AnimationGear v7 (Autodesk Fusion 360 design; units mm, degrees)
Autodesk Fusion 360 part; units mm, degrees
note: some values were not read from the file. Set by a fixed rule: which sketch regions a step uses.
sketch "Sketch1" plane through (0, 0, 0) normal (0, 1, 0) x (1, 0, 0)
  line L0 (7.1438, 0) -> (11.7891, 0)
  line L1 (11.7891, 0) -> (11.8321, 0.0026)
  line L2 (11.8321, 0.0026) -> (11.9318, 0.0152)
  line L3 (11.9318, 0.0152) -> (12.0868, 0.0457)
  line L4 (12.0868, 0.0457) -> (12.2948, 0.1017)
  line L5 (12.2948, 0.1017) -> (12.5526, 0.1909)
  line L6 (12.5526, 0.1909) -> (12.8565, 0.3202)
  line L7 (12.8565, 0.3202) -> (13.2018, 0.4965)
  line L8 (13.2018, 0.4965) -> (13.5832, 0.7261)
  line L9 (13.5832, 0.7261) -> (13.9947, 1.0146)
  line L10 (13.9947, 1.0146) -> (14.4297, 1.3673)
  line L11 (14.4297, 1.3673) -> (14.881, 1.7887)
  line L12 (14.881, 1.7887) -> (15.3411, 2.2825)
  line L13 (15.3411, 2.2825) -> (15.8017, 2.8518)
  line L14 (15.8017, 2.8518) -> (16.2544, 3.499)
  line L15 (16.2544, 3.499) -> (16.6905, 4.2253)
  line L16 (16.6905, 4.2253) -> (17.1009, 5.0316)
  line L17 (17.1009, 5.0316) -> (17.4765, 5.9173)
  line L18 (17.4765, 5.9173) -> (17.1551, 6.7931)
  line L19 (17.1551, 6.7931) -> (16.2957, 7.2255)
  line L20 (16.2957, 7.2255) -> (15.4612, 7.5748)
  line L21 (15.4612, 7.5748) -> (14.6587, 7.8467)
  line L22 (14.6587, 7.8467) -> (13.8949, 8.0473)
  line L23 (13.8949, 8.0473) -> (13.1753, 8.1835)
  line L24 (13.1753, 8.1835) -> (12.5051, 8.2625)
  line L25 (12.5051, 8.2625) -> (11.8883, 8.2918)
  line L26 (11.8883, 8.2918) -> (11.3284, 8.2793)
  line L27 (11.3284, 8.2793) -> (10.828, 8.2332)
  line L28 (10.828, 8.2332) -> (10.3886, 8.1615)
  line L29 (10.3886, 8.1615) -> (10.0113, 8.0726)
  line L30 (10.0113, 8.0726) -> (9.6958, 7.9747)
  line L31 (9.6958, 7.9747) -> (9.4415, 7.8758)
  line L32 (9.4415, 7.8758) -> (9.2467, 7.7841)
  line L33 (9.2467, 7.7841) -> (9.1088, 7.707)
  line L34 (9.1088, 7.707) -> (9.0246, 7.6521)
  line L35 (9.0246, 7.6521) -> (8.9901, 7.6263)
  line L36 (8.9901, 7.6263) -> (5.4477, 4.6213)
  line L37 (5.4477, 4.6213) -> (2.2076, 6.7941)
  line L38 (2.2076, 6.7941) -> (3.643, 11.2121)
  line L39 (3.643, 11.2121) -> (3.6538, 11.2538)
  line L40 (3.6538, 11.2538) -> (3.6727, 11.3525)
  line L41 (3.6727, 11.3525) -> (3.6916, 11.5093)
  line L42 (3.6916, 11.5093) -> (3.7025, 11.7244)
  line L43 (3.7025, 11.7244) -> (3.6974, 11.9972)
  line L44 (3.6974, 11.9972) -> (3.6683, 12.3262)
  line L45 (3.6683, 12.3262) -> (3.6074, 12.7091)
  line L46 (3.6074, 12.7091) -> (3.5069, 13.1428)
  line L47 (3.5069, 13.1428) -> (3.3596, 13.6233)
  line L48 (3.3596, 13.6233) -> (3.1586, 14.146)
  line L49 (3.1586, 14.146) -> (2.8974, 14.7054)
  line L50 (2.8974, 14.7054) -> (2.5699, 15.2956)
  line L51 (2.5699, 15.2956) -> (2.1707, 15.9096)
  line L52 (2.1707, 15.9096) -> (1.6952, 16.5401)
  line L53 (1.6952, 16.5401) -> (1.1391, 17.1793)
  line L54 (1.1391, 17.1793) -> (0.4992, 17.8187)
  line L55 (0.4992, 17.8187) -> (-0.2271, 18.4497)
  line L56 (-0.2271, 18.4497) -> (-1.1594, 18.4146)
  line L57 (-1.1594, 18.4146) -> (-1.8362, 17.7309)
  line L58 (-1.8362, 17.7309) -> (-2.4263, 17.0452)
  line L59 (-2.4263, 17.0452) -> (-2.9328, 16.366)
  line L60 (-2.9328, 16.366) -> (-3.3597, 15.7016)
  line L61 (-3.3597, 15.7016) -> (-3.7115, 15.0593)
  line L62 (-3.7115, 15.0593) -> (-3.9938, 14.4463)
  line L63 (-3.9938, 14.4463) -> (-4.2123, 13.8687)
  line L64 (-4.2123, 13.8687) -> (-4.3735, 13.3324)
  line L65 (-4.3735, 13.3324) -> (-4.4842, 12.8422)
  line L66 (-4.4842, 12.8422) -> (-4.5518, 12.4022)
  line L67 (-4.5518, 12.4022) -> (-4.5839, 12.0158)
  line L68 (-4.5839, 12.0158) -> (-4.5882, 11.6856)
  line L69 (-4.5882, 11.6856) -> (-4.5728, 11.4132)
  line L70 (-4.5728, 11.4132) -> (-4.5457, 11.1995)
  line L71 (-4.5457, 11.1995) -> (-4.5151, 11.0446)
  line L72 (-4.5151, 11.0446) -> (-4.4888, 10.9475)
  line L73 (-4.4888, 10.9475) -> (-4.4749, 10.9068)
  line L74 (-4.4749, 10.9068) -> (-2.7117, 6.6091)
  line L75 (-2.7117, 6.6091) -> (-5.7794, 4.199)
  line L76 (-5.7794, 4.199) -> (-9.5376, 6.9294)
  line L77 (-9.5376, 6.9294) -> (-9.5739, 6.9526)
  line L78 (-9.5739, 6.9526) -> (-9.6619, 7.001)
  line L79 (-9.6619, 7.001) -> (-9.8052, 7.0675)
  line L80 (-9.8052, 7.0675) -> (-10.0065, 7.1444)
  line L81 (-10.0065, 7.1444) -> (-10.2675, 7.2238)
  line L82 (-10.2675, 7.2238) -> (-10.5893, 7.2978)
  line L83 (-10.5893, 7.2978) -> (-10.9723, 7.3581)
  line L84 (-10.9723, 7.3581) -> (-11.4158, 7.3966)
  line L85 (-11.4158, 7.3966) -> (-11.9183, 7.405)
  line L86 (-11.9183, 7.405) -> (-12.4776, 7.3754)
  line L87 (-12.4776, 7.3754) -> (-13.0904, 7.2998)
  line L88 (-13.0904, 7.2998) -> (-13.7528, 7.1707)
  line L89 (-13.7528, 7.1707) -> (-14.4601, 6.9808)
  line L90 (-14.4601, 6.9808) -> (-15.2067, 6.7234)
  line L91 (-15.2067, 6.7234) -> (-15.9865, 6.392)
  line L92 (-15.9865, 6.392) -> (-16.7924, 5.981)
  line L93 (-16.7924, 5.981) -> (-17.6169, 5.4852)
  line L94 (-17.6169, 5.4852) -> (-17.8716, 4.5878)
  line L95 (-17.8716, 4.5878) -> (-17.4305, 3.7328)
  line L96 (-17.4305, 3.7328) -> (-16.9607, 2.9597)
  line L97 (-16.9607, 2.9597) -> (-16.4713, 2.2681)
  line L98 (-16.4713, 2.2681) -> (-15.9713, 1.6568)
  line L99 (-15.9713, 1.6568) -> (-15.4692, 1.1237)
  line L100 (-15.4692, 1.1237) -> (-14.9734, 0.6658)
  line L101 (-14.9734, 0.6658) -> (-14.4916, 0.2796)
  line L102 (-14.4916, 0.2796) -> (-14.0314, -0.0395)
  line L103 (-14.0314, -0.0395) -> (-13.5993, -0.2963)
  line L104 (-13.5993, -0.2963) -> (-13.2018, -0.4965)
  line L105 (-13.2018, -0.4965) -> (-12.8442, -0.6464)
  line L106 (-12.8442, -0.6464) -> (-12.5315, -0.7526)
  line L107 (-12.5315, -0.7526) -> (-12.2677, -0.8221)
  line L108 (-12.2677, -0.8221) -> (-12.0561, -0.8624)
  line L109 (-12.0561, -0.8624) -> (-11.8992, -0.8811)
  line L110 (-11.8992, -0.8811) -> (-11.7988, -0.8862)
  line L111 (-11.7988, -0.8862) -> (-11.7558, -0.8855)
  line L112 (-11.7558, -0.8855) -> (-7.1236, -0.5366)
  line L113 (-7.1236, -0.5366) -> (-5.7794, -4.199)
  line L114 (-5.7794, -4.199) -> (-9.5375, -6.9295)
  line L115 (-9.5375, -6.9295) -> (-9.5708, -6.9568)
  line L116 (-9.5708, -6.9568) -> (-9.6441, -7.0256)
  line L117 (-9.6441, -7.0256) -> (-9.7516, -7.1414)
  line L118 (-9.7516, -7.1414) -> (-9.8869, -7.309)
  line L119 (-9.8869, -7.309) -> (-10.0431, -7.5327)
  line L120 (-10.0431, -7.5327) -> (-10.2129, -7.8159)
  line L121 (-10.2129, -7.8159) -> (-10.3886, -8.1615)
  line L122 (-10.3886, -8.1615) -> (-10.5622, -8.5714)
  line L123 (-10.5622, -8.5714) -> (-10.7255, -9.0467)
  line L124 (-10.7255, -9.0467) -> (-10.8702, -9.5878)
  line L125 (-10.8702, -9.5878) -> (-10.9877, -10.1939)
  line L126 (-10.9877, -10.1939) -> (-11.0696, -10.8638)
  line L127 (-11.0696, -10.8638) -> (-11.1076, -11.5952)
  line L128 (-11.1076, -11.5952) -> (-11.0935, -12.3848)
  line L129 (-11.0935, -12.3848) -> (-11.0193, -13.2288)
  line L130 (-11.0193, -13.2288) -> (-10.8774, -14.1222)
  line L131 (-10.8774, -14.1222) -> (-10.6607, -15.0596)
  line L132 (-10.6607, -15.0596) -> (-9.8859, -15.5792)
  line L133 (-9.8859, -15.5792) -> (-8.9364, -15.4239)
  line L134 (-8.9364, -15.4239) -> (-8.056, -15.216)
  line L135 (-8.056, -15.216) -> (-7.247, -14.9643)
  line L136 (-7.247, -14.9643) -> (-6.5111, -14.6776)
  line L137 (-6.5111, -14.6776) -> (-5.8489, -14.3648)
  line L138 (-5.8489, -14.3648) -> (-5.2603, -14.0348)
  line L139 (-5.2603, -14.0348) -> (-4.744, -13.696)
  line L140 (-4.744, -13.696) -> (-4.2984, -13.3568)
  line L141 (-4.2984, -13.3568) -> (-3.9206, -13.0253)
  line L142 (-3.9206, -13.0253) -> (-3.6074, -12.7091)
  line L143 (-3.6074, -12.7091) -> (-3.3543, -12.4153)
  line L144 (-3.3543, -12.4153) -> (-3.1567, -12.1507)
  line L145 (-3.1567, -12.1507) -> (-3.0091, -11.9213)
  line L146 (-3.0091, -11.9213) -> (-2.9054, -11.7325)
  line L147 (-2.9054, -11.7325) -> (-2.8391, -11.5891)
  line L148 (-2.8391, -11.5891) -> (-2.8032, -11.4952)
  line L149 (-2.8032, -11.4952) -> (-2.7905, -11.4541)
  line L150 (-2.7905, -11.4541) -> (-1.691, -6.9407)
  line L151 (-1.691, -6.9407) -> (2.2076, -6.7941)
  line L152 (2.2076, -6.7941) -> (3.643, -11.2121)
  line L153 (3.643, -11.2121) -> (3.6588, -11.2522)
  line L154 (3.6588, -11.2522) -> (3.7016, -11.3431)
  line L155 (3.7016, -11.3431) -> (3.7784, -11.4811)
  line L156 (3.7784, -11.4811) -> (3.896, -11.6616)
  line L157 (3.896, -11.6616) -> (4.0605, -11.8793)
  line L158 (4.0605, -11.8793) -> (4.2774, -12.1283)
  line L159 (4.2774, -12.1283) -> (4.5518, -12.4022)
  line L160 (4.5518, -12.4022) -> (4.888, -12.694)
  line L161 (4.888, -12.694) -> (5.2896, -12.9962)
  line L162 (5.2896, -12.9962) -> (5.7594, -13.3009)
  line L163 (5.7594, -13.3009) -> (6.2996, -13.6)
  line L164 (6.2996, -13.6) -> (6.9114, -13.8849)
  line L165 (6.9114, -13.8849) -> (7.5953, -14.147)
  line L166 (7.5953, -14.147) -> (8.3506, -14.3776)
  line L167 (8.3506, -14.3776) -> (9.1762, -14.5679)
  line L168 (9.1762, -14.5679) -> (10.0698, -14.7091)
  line L169 (10.0698, -14.7091) -> (11.0282, -14.7926)
  line L170 (11.0282, -14.7926) -> (11.7618, -14.2163)
  line L171 (11.7618, -14.2163) -> (11.9075, -13.2653)
  line L172 (11.9075, -13.2653) -> (11.9818, -12.3637)
  line L173 (11.9818, -12.3637) -> (11.9924, -11.5165)
  line L174 (11.9924, -11.5165) -> (11.9472, -10.7281)
  line L175 (11.9472, -10.7281) -> (11.8544, -10.0016)
  line L176 (11.8544, -10.0016) -> (11.7223, -9.3398)
  line L177 (11.7223, -9.3398) -> (11.5596, -8.7441)
  line L178 (11.5596, -8.7441) -> (11.3748, -8.2155)
  line L179 (11.3748, -8.2155) -> (11.1763, -7.7538)
  line L180 (11.1763, -7.7538) -> (10.9723, -7.3581)
  line L181 (10.9723, -7.3581) -> (10.7712, -7.0267)
  line L182 (10.7712, -7.0267) -> (10.5805, -6.757)
  line L183 (10.5805, -6.757) -> (10.408, -6.5457)
  line L184 (10.408, -6.5457) -> (10.2605, -6.3887)
  line L185 (10.2605, -6.3887) -> (10.1446, -6.2813)
  line L186 (10.1446, -6.2813) -> (10.0663, -6.2182)
  line L187 (10.0663, -6.2182) -> (10.0311, -6.1934)
  line L188 (10.0311, -6.1934) -> (6.0785, -3.753)
  line L189 (6.0785, -3.753) -> (7.1438, 0)
  line L190 (2.6458, 0) -> (-2.6458, 0)
  line L191 (0, -2.6458) -> (0, 2.6458)
  circle A0 centre (12.4191, 4.558) radius 2.077
  circle A1 centre (0, 0) radius 13.2292
  circle A2 centre (0, 0) radius 18.5208
  circle A3 centre (0, 0) radius 11.7872
  circle A4 centre (0, 0) radius 1.5
  dimension "d1" = 3
  constraint concentric A2 A4
  measures "d1" diameter of A4
extrude "Extrude1" add sketch "Sketch1" along normal blind 5 contours L0 L36 L37 L38 L74 L75 L76 L112 L113 L114 L150 L151 L152 L188 L189 A0 A3 | L1 L2 L3 L4 L5 L6 L7 L8 A0 A1 A3 | L153 L154 L155 L156 L157 L158 L159 L160 L180 L181 L182 L183 L184 L185 L186 L187 A1 A3 | A0 A1 A3 | A0 A3 | L28 L29 L30 L31 L32 L33 L34 L35 A0 A1 A3 | A0 A1 | L8 L9 L10 L11 L12 L13 L14 L15 L16 L17 L18 L19 L20 L21 L22 L23 L24 L25 L26 L27 L28 A0 A1 | L115 L116 L117 L118 L119 L120 L121 L122 L142 L143 L144 L145 L146 L147 L148 L149 A1 A3 | L39 L40 L41 L42 L43 L44 L45 L46 L66 L67 L68 L69 L70 L71 L72 L73 A1 A3 | L77 L78 L79 L80 L81 L82 L83 L84 L104 L105 L106 L107 L108 L109 L110 L111 A1 A3 | L46 L47 L48 L49 L50 L51 L52 L53 L54 L55 L56 L57 L58 L59 L60 L61 L62 L63 L64 L65 L66 A1 | L160 L161 L162 L163 L164 L165 L166 L167 L168 L169 L170 L171 L172 L173 L174 L175 L176 L177 L178 L179 L180 A1 | L84 L85 L86 L87 L88 L89 L90 L91 L92 L93 L94 L95 L96 L97 L98 L99 L100 L101 L102 L103 L104 A1 | L122 L123 L124 L125 L126 L127 L128 L129 L130 L131 L132 L133 L134 L135 L136 L137 L138 L139 L140 L141 L142 A1
sketch "Sketch2" plane through (0, 5, 0) normal (0, 1, 0) x (-1, 0, 0)
  circle A0 centre (0, 0) radius 1.5
  line L0 (-6.0785, 3.753) -> (-7.1438, 0)
  line L1 (-7.1438, 0) -> (-11.7891, 0)
  line L2 (-11.7891, 0) -> (-11.8321, -0.0026)
  line L3 (-11.8321, -0.0026) -> (-11.9318, -0.0152)
  line L4 (-11.9318, -0.0152) -> (-12.0868, -0.0457)
  line L5 (-12.0868, -0.0457) -> (-12.2948, -0.1017)
  line L6 (-12.2948, -0.1017) -> (-12.5526, -0.1909)
  line L7 (-12.5526, -0.1909) -> (-12.8565, -0.3202)
  line L8 (-12.8565, -0.3202) -> (-13.2018, -0.4965)
  line L9 (-13.2018, -0.4965) -> (-13.5832, -0.7261)
  line L10 (-13.5832, -0.7261) -> (-13.9947, -1.0146)
  line L11 (-13.9947, -1.0146) -> (-14.4297, -1.3673)
  line L12 (-14.4297, -1.3673) -> (-14.881, -1.7887)
  line L13 (-14.881, -1.7887) -> (-15.3411, -2.2825)
  line L14 (-15.3411, -2.2825) -> (-15.8017, -2.8518)
  line L15 (-15.8017, -2.8518) -> (-16.2544, -3.499)
  line L16 (-16.2544, -3.499) -> (-16.6905, -4.2253)
  line L17 (-16.6905, -4.2253) -> (-17.1009, -5.0316)
  line L18 (-17.1009, -5.0316) -> (-17.4765, -5.9173)
  line L19 (-17.4765, -5.9173) -> (-17.1551, -6.7931)
  line L20 (-17.1551, -6.7931) -> (-16.2957, -7.2255)
  line L21 (-16.2957, -7.2255) -> (-15.4612, -7.5748)
  line L22 (-15.4612, -7.5748) -> (-14.6587, -7.8467)
  line L23 (-14.6587, -7.8467) -> (-13.8949, -8.0473)
  line L24 (-13.8949, -8.0473) -> (-13.1753, -8.1835)
  line L25 (-13.1753, -8.1835) -> (-12.5051, -8.2625)
  line L26 (-12.5051, -8.2625) -> (-11.8883, -8.2918)
  line L27 (-11.8883, -8.2918) -> (-11.3284, -8.2793)
  line L28 (-11.3284, -8.2793) -> (-10.828, -8.2332)
  line L29 (-10.828, -8.2332) -> (-10.3886, -8.1615)
  line L30 (-10.3886, -8.1615) -> (-10.0113, -8.0726)
  line L31 (-10.0113, -8.0726) -> (-9.6958, -7.9747)
  line L32 (-9.6958, -7.9747) -> (-9.4415, -7.8758)
  line L33 (-9.4415, -7.8758) -> (-9.2467, -7.7841)
  line L34 (-9.2467, -7.7841) -> (-9.1088, -7.707)
  line L35 (-9.1088, -7.707) -> (-9.0246, -7.6521)
  line L36 (-9.0246, -7.6521) -> (-8.9901, -7.6263)
  line L37 (-8.9901, -7.6263) -> (-5.4477, -4.6213)
  line L38 (-5.4477, -4.6213) -> (-2.2076, -6.7941)
  line L39 (-2.2076, -6.7941) -> (-3.643, -11.2121)
  line L40 (-3.643, -11.2121) -> (-3.6538, -11.2538)
  line L41 (-3.6538, -11.2538) -> (-3.6727, -11.3525)
  line L42 (-3.6727, -11.3525) -> (-3.6916, -11.5093)
  line L43 (-3.6916, -11.5093) -> (-3.7025, -11.7244)
  line L44 (-3.7025, -11.7244) -> (-3.6974, -11.9972)
  line L45 (-3.6974, -11.9972) -> (-3.6683, -12.3262)
  line L46 (-3.6683, -12.3262) -> (-3.6074, -12.7091)
  line L47 (-3.6074, -12.7091) -> (-3.5069, -13.1428)
  line L48 (-3.5069, -13.1428) -> (-3.3596, -13.6233)
  line L49 (-3.3596, -13.6233) -> (-3.1586, -14.146)
  line L50 (-3.1586, -14.146) -> (-2.8974, -14.7054)
  line L51 (-2.8974, -14.7054) -> (-2.5699, -15.2956)
  line L52 (-2.5699, -15.2956) -> (-2.1707, -15.9096)
  line L53 (-2.1707, -15.9096) -> (-1.6952, -16.5401)
  line L54 (-1.6952, -16.5401) -> (-1.1391, -17.1793)
  line L55 (-1.1391, -17.1793) -> (-0.4992, -17.8187)
  line L56 (-0.4992, -17.8187) -> (0.2271, -18.4497)
  line L57 (0.2271, -18.4497) -> (1.1594, -18.4146)
  line L58 (1.1594, -18.4146) -> (1.8362, -17.7309)
  line L59 (1.8362, -17.7309) -> (2.4263, -17.0452)
  line L60 (2.4263, -17.0452) -> (2.9328, -16.366)
  line L61 (2.9328, -16.366) -> (3.3597, -15.7016)
  line L62 (3.3597, -15.7016) -> (3.7115, -15.0593)
  line L63 (3.7115, -15.0593) -> (3.9938, -14.4463)
  line L64 (3.9938, -14.4463) -> (4.2123, -13.8687)
  line L65 (4.2123, -13.8687) -> (4.3735, -13.3324)
  line L66 (4.3735, -13.3324) -> (4.4842, -12.8422)
  line L67 (4.4842, -12.8422) -> (4.5518, -12.4022)
  line L68 (4.5518, -12.4022) -> (4.5839, -12.0158)
  line L69 (4.5839, -12.0158) -> (4.5882, -11.6856)
  line L70 (4.5882, -11.6856) -> (4.5728, -11.4132)
  line L71 (4.5728, -11.4132) -> (4.5457, -11.1995)
  line L72 (4.5457, -11.1995) -> (4.5151, -11.0446)
  line L73 (4.5151, -11.0446) -> (4.4888, -10.9475)
  line L74 (4.4888, -10.9475) -> (4.4749, -10.9068)
  line L75 (4.4749, -10.9068) -> (2.7117, -6.6091)
  line L76 (2.7117, -6.6091) -> (5.7794, -4.199)
  line L77 (5.7794, -4.199) -> (9.5376, -6.9294)
  line L78 (9.5376, -6.9294) -> (9.5739, -6.9526)
  line L79 (9.5739, -6.9526) -> (9.6619, -7.001)
  line L80 (9.6619, -7.001) -> (9.8052, -7.0675)
  line L81 (9.8052, -7.0675) -> (10.0065, -7.1444)
  line L82 (10.0065, -7.1444) -> (10.2675, -7.2238)
  line L83 (10.2675, -7.2238) -> (10.5893, -7.2978)
  line L84 (10.5893, -7.2978) -> (10.9723, -7.3581)
  line L85 (10.9723, -7.3581) -> (11.4158, -7.3966)
  line L86 (11.4158, -7.3966) -> (11.9183, -7.405)
  line L87 (11.9183, -7.405) -> (12.4776, -7.3754)
  line L88 (12.4776, -7.3754) -> (13.0904, -7.2998)
  line L89 (13.0904, -7.2998) -> (13.7528, -7.1707)
  line L90 (13.7528, -7.1707) -> (14.4601, -6.9808)
  line L91 (14.4601, -6.9808) -> (15.2067, -6.7234)
  line L92 (15.2067, -6.7234) -> (15.9865, -6.392)
  line L93 (15.9865, -6.392) -> (16.7924, -5.981)
  line L94 (16.7924, -5.981) -> (17.6169, -5.4852)
  line L95 (17.6169, -5.4852) -> (17.8716, -4.5878)
  line L96 (17.8716, -4.5878) -> (17.4305, -3.7328)
  line L97 (17.4305, -3.7328) -> (16.9607, -2.9597)
  line L98 (16.9607, -2.9597) -> (16.4713, -2.2681)
  line L99 (16.4713, -2.2681) -> (15.9713, -1.6568)
  line L100 (15.9713, -1.6568) -> (15.4692, -1.1237)
  line L101 (15.4692, -1.1237) -> (14.9734, -0.6658)
  line L102 (14.9734, -0.6658) -> (14.4916, -0.2796)
  line L103 (14.4916, -0.2796) -> (14.0314, 0.0395)
  line L104 (14.0314, 0.0395) -> (13.5993, 0.2963)
  line L105 (13.5993, 0.2963) -> (13.2018, 0.4965)
  line L106 (13.2018, 0.4965) -> (12.8442, 0.6464)
  line L107 (12.8442, 0.6464) -> (12.5315, 0.7526)
  line L108 (12.5315, 0.7526) -> (12.2677, 0.8221)
  line L109 (12.2677, 0.8221) -> (12.0561, 0.8624)
  line L110 (12.0561, 0.8624) -> (11.8992, 0.8811)
  line L111 (11.8992, 0.8811) -> (11.7988, 0.8862)
  line L112 (11.7988, 0.8862) -> (11.7558, 0.8855)
  line L113 (11.7558, 0.8855) -> (7.1236, 0.5366)
  line L114 (7.1236, 0.5366) -> (5.7794, 4.199)
  line L115 (5.7794, 4.199) -> (9.5375, 6.9295)
  line L116 (9.5375, 6.9295) -> (9.5708, 6.9568)
  line L117 (9.5708, 6.9568) -> (9.6441, 7.0256)
  line L118 (9.6441, 7.0256) -> (9.7516, 7.1414)
  line L119 (9.7516, 7.1414) -> (9.8869, 7.309)
  line L120 (9.8869, 7.309) -> (10.0431, 7.5327)
  line L121 (10.0431, 7.5327) -> (10.2129, 7.8159)
  line L122 (10.2129, 7.8159) -> (10.3886, 8.1615)
  line L123 (10.3886, 8.1615) -> (10.5622, 8.5714)
  line L124 (10.5622, 8.5714) -> (10.7255, 9.0467)
  line L125 (10.7255, 9.0467) -> (10.8702, 9.5878)
  line L126 (10.8702, 9.5878) -> (10.9877, 10.1939)
  line L127 (10.9877, 10.1939) -> (11.0696, 10.8638)
  line L128 (11.0696, 10.8638) -> (11.1076, 11.5952)
  line L129 (11.1076, 11.5952) -> (11.0935, 12.3848)
  line L130 (11.0935, 12.3848) -> (11.0193, 13.2288)
  line L131 (11.0193, 13.2288) -> (10.8774, 14.1222)
  line L132 (10.8774, 14.1222) -> (10.6607, 15.0596)
  line L133 (10.6607, 15.0596) -> (9.8859, 15.5792)
  line L134 (9.8859, 15.5792) -> (8.9364, 15.4239)
  line L135 (8.9364, 15.4239) -> (8.056, 15.216)
  line L136 (8.056, 15.216) -> (7.247, 14.9643)
  line L137 (7.247, 14.9643) -> (6.5111, 14.6776)
  line L138 (6.5111, 14.6776) -> (5.8489, 14.3648)
  line L139 (5.8489, 14.3648) -> (5.2603, 14.0348)
  line L140 (5.2603, 14.0348) -> (4.744, 13.696)
  line L141 (4.744, 13.696) -> (4.2984, 13.3568)
  line L142 (4.2984, 13.3568) -> (3.9206, 13.0253)
  line L143 (3.9206, 13.0253) -> (3.6074, 12.7091)
  line L144 (3.6074, 12.7091) -> (3.3543, 12.4153)
  line L145 (3.3543, 12.4153) -> (3.1567, 12.1507)
  line L146 (3.1567, 12.1507) -> (3.0091, 11.9213)
  line L147 (3.0091, 11.9213) -> (2.9054, 11.7325)
  line L148 (2.9054, 11.7325) -> (2.8391, 11.5891)
  line L149 (2.8391, 11.5891) -> (2.8032, 11.4952)
  line L150 (2.8032, 11.4952) -> (2.7905, 11.4541)
  line L151 (2.7905, 11.4541) -> (1.691, 6.9407)
  line L152 (1.691, 6.9407) -> (-2.2076, 6.7941)
  line L153 (-2.2076, 6.7941) -> (-3.643, 11.2121)
  line L154 (-3.643, 11.2121) -> (-3.6588, 11.2522)
  line L155 (-3.6588, 11.2522) -> (-3.7016, 11.3431)
  line L156 (-3.7016, 11.3431) -> (-3.7784, 11.4811)
  line L157 (-3.7784, 11.4811) -> (-3.896, 11.6616)
  line L158 (-3.896, 11.6616) -> (-4.0605, 11.8793)
  line L159 (-4.0605, 11.8793) -> (-4.2774, 12.1283)
  line L160 (-4.2774, 12.1283) -> (-4.5518, 12.4022)
  line L161 (-4.5518, 12.4022) -> (-4.888, 12.694)
  line L162 (-4.888, 12.694) -> (-5.2896, 12.9962)
  line L163 (-5.2896, 12.9962) -> (-5.7594, 13.3009)
  line L164 (-5.7594, 13.3009) -> (-6.2996, 13.6)
  line L165 (-6.2996, 13.6) -> (-6.9114, 13.8849)
  line L166 (-6.9114, 13.8849) -> (-7.5953, 14.147)
  line L167 (-7.5953, 14.147) -> (-8.3506, 14.3776)
  line L168 (-8.3506, 14.3776) -> (-9.1762, 14.5679)
  line L169 (-9.1762, 14.5679) -> (-10.0698, 14.7091)
  line L170 (-10.0698, 14.7091) -> (-11.0282, 14.7926)
  line L171 (-11.0282, 14.7926) -> (-11.7618, 14.2163)
  line L172 (-11.7618, 14.2163) -> (-11.9075, 13.2653)
  line L173 (-11.9075, 13.2653) -> (-11.9818, 12.3637)
  line L174 (-11.9818, 12.3637) -> (-11.9924, 11.5165)
  line L175 (-11.9924, 11.5165) -> (-11.9472, 10.7281)
  line L176 (-11.9472, 10.7281) -> (-11.8544, 10.0016)
  line L177 (-11.8544, 10.0016) -> (-11.7223, 9.3398)
  line L178 (-11.7223, 9.3398) -> (-11.5596, 8.7441)
  line L179 (-11.5596, 8.7441) -> (-11.3748, 8.2155)
  line L180 (-11.3748, 8.2155) -> (-11.1763, 7.7538)
  line L181 (-11.1763, 7.7538) -> (-10.9723, 7.3581)
  line L182 (-10.9723, 7.3581) -> (-10.7712, 7.0267)
  line L183 (-10.7712, 7.0267) -> (-10.5805, 6.757)
  line L184 (-10.5805, 6.757) -> (-10.408, 6.5457)
  line L185 (-10.408, 6.5457) -> (-10.2605, 6.3887)
  line L186 (-10.2605, 6.3887) -> (-10.1446, 6.2813)
  line L187 (-10.1446, 6.2813) -> (-10.0663, 6.2182)
  line L188 (-10.0663, 6.2182) -> (-10.0311, 6.1934)
  line L189 (-10.0311, 6.1934) -> (-6.0785, 3.753)
  line L190 (-17.3158, -6.3552) -> (0, 0) construction
  line L191 (0, 0) -> (-4.6939, -1.7227)
  circle A1 centre (-4.6939, -1.7227) radius 1.5
  dimension "d4" = 5
  dimension "d5" = 3
  constraint midpoint L19 A0.centre
  constraint coincident A0.centre L190.end
  constraint coincident L190 A0.centre
  measures "d5" diameter of A1
extrude "Extrude2" add sketch "Sketch2" along normal blind 3 contours A1
